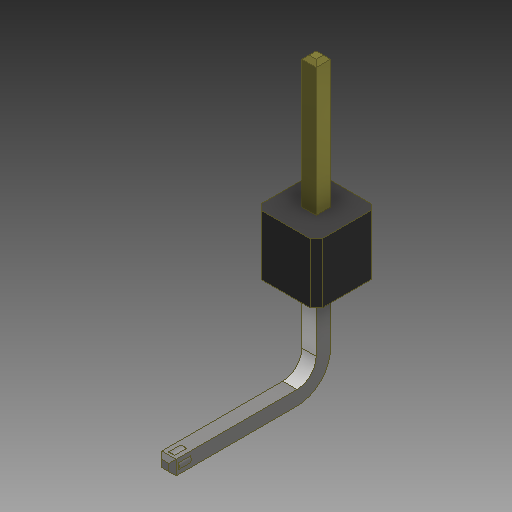
# Autodesk Inventor part: Stiftleiste_Male_90
Saved by Autodesk Inventor 2017 SP1 (Build 210196100, 196)
## iProperties
Part Number: Stiftleiste_Male_90
Material: Generisch
Document SubType Name: Modeling
Designer: Alex
Density: 1 g/cm^3
Appearance: Vorgabe2
Author: Alex
Autodesk Inventor part; units mm, degrees
ref_plane "YZ Plane" through (0, 0, 0) normal (1, 0, 0) x (0, 1, 0)
sketch "Skizze2" plane through (0, 0, 0) normal (0, 0, 1) x (1, 0, 0)
  line L0 (0, 0) -> (-0.6, 0)
  line L1 (-0.6, 0) -> (-0.6, 0.6)
  line L2 (-0.6, 0.6) -> (0, 0.6)
  line L3 (0, 0.6) -> (0, 0)
  dimension "d0" = 0.6
  dimension "d1" = 0.6
  constraints: 8 end point, 2 parallel, 1 horizontal, 1 perpendicular
  measures "d0" distance of L1.end L2.end
  measures "d1" distance of L0.end L1.end
extrude "Extrusion1" add sketch "Skizze2" along normal blind 11
ref_plane "Arbeitsebene1" through (0, 0, 3) normal (0, 0, -1) x (-1, 0, 0)
sketch "Skizze3" plane through (0, 0, 3) normal (0, 0, -1) x (-1, 0, 0)
  line L0 (1.57, 1.57) -> (-0.97, 1.57)
  line L1 (-0.97, 1.57) -> (-0.97, -0.97)
  line L2 (-0.97, -0.97) -> (1.57, -0.97)
  line L3 (1.57, -0.97) -> (1.57, 1.57)
  line L4 (0.6, 0) -> (0.6, 0.6) projected
  line L5 (0, 0.6) -> (0.6, 0.6) projected
  point P0 (0, 0)
  dimension "d5" = 2.54
  dimension "d6" = 2.54
  dimension "d7" = 0.97
  dimension "d8" = 0.97
  constraints: 8 end point, 2 parallel, 1 horizontal, 1 perpendicular
  measures "d5" distance of L2.end L1.end
  measures "d6" distance of L1.end L0.end
  measures "d7" distance between parallel lines of L4 L3
  measures "d8" distance between parallel lines of L0 L5
extrude "Extrusion2" add sketch "Skizze3" against normal blind 2.5
chamfer "Fase1" distance 0.25 angle 45 4 edges at (0.97, -0.97, 4.25) (-1.57, -0.97, 4.25) (-1.57, 1.57, 4.25) (0.97, 1.57, 4.25)
sketch "Skizze6" plane through (0, 0, 0) normal (0, 0, -1) x (-1, 0, 0)
  line L0 (0, 0.6) -> (0, 0) projected
  line L1 (0, 0.6) -> (0.6, 0.6)
  line L2 (0.6, 0.6) -> (0.6, 0)
  line L3 (0.6, 0) -> (0, 0)
  line L4 (0, 0) -> (0, 0.6)
  constraints: 8 end point, 2 parallel, 1 horizontal, 1 perpendicular
extrude "Extrusion4" add sketch "Skizze6" along normal blind 1
sketch "Skizze7" plane through (-0.6, 0, 3) normal (0, -1, 0) x (1, 0, 0)
  line L0 (0.6, -4) -> (0, -4) projected
  line L1 (0.6, -4) -> (0, -4)
  line L2 (0, -4) -> (0, -3.4)
  line L3 (0, -3.4) -> (0.6, -3.4)
  line L4 (0.6, -3.4) -> (0.6, -4)
  point P0 (0.6, -3)
  dimension "d27" = 0.6
  constraints: 8 end point, 2 parallel, 1 horizontal, 1 perpendicular
  measures "d27" distance of L1.end L2.end
extrude "Extrusion5" add sketch "Skizze7" along normal blind 6
chamfer "Fase3" distance 0.15 angle 45 8 edges at (-0.6, 0.3, 11) (-0.3, 0, 11) (0, 0.3, 11) (-0.3, 0.6, 11) (0, -6, -0.7) (-0.3, -6, -0.4) (-0.6, -6, -0.7) (-0.3, -6, -1)
fillet "Rundung1" radius 0.8 1 edges at (-0.3, 0, -0.4)
fillet "Rundung2" radius 1.4 1 edges at (-0.3, 0.6, -1)
ref_plane "Arbeitsebene2" through (-0.6, -5.75, 3) normal (0, -1, 0) x (1, 0, 0)
sketch "Skizze8" plane through (-0.6, -5.75, 3) normal (0, -1, 0) x (1, 0, 0)
  circle A0 centre (0.3, -3.7) radius 0.325
  line L0 (0, -4) -> (0.6, -4) projected
  line L1 (0, -3.4) -> (0, -4) projected
  point P0 (0.6, -3)
  dimension "d33" = 0.65
  dimension "d34" = 0.3
  dimension "d35" = 0.3
  constraints: 1 centre point
  measures "d33" diameter of A0
  measures "d34" distance from line of L0 A0.centre
  measures "d35" distance from line of L1 A0.centre
extrude "Extrusion6" add sketch "Skizze8" against normal blind 0.5 contours A0 L0 L1 | L1 A0 | A0 L0 picked at (0.321, -3.7679)
